Autodesk Inventor part; units mm, degrees
(part 2 of 2)
sketch "Sketch_56" plane through (0, -45.7, 0) normal (0, 1, 0) x (1, 0, 0)
  line L0 (-9.05, 22.27) -> (-9.05, 19.07)
  arc A0 (-9.05, 19.07) -> (-8.65, 18.67) centre (-8.65, 19.07) ccw
  line L1 (-8.65, 18.67) -> (-5.25, 18.67)
  line L2 (-5.25, 18.67) -> (-5.25, 20.67)
  line L3 (-5.25, 20.67) -> (-7.45, 20.67)
  line L4 (-7.45, 20.67) -> (-7.45, 21.67)
  line L5 (-7.45, 21.67) -> (-8.05, 22.67)
  line L6 (-8.05, 22.67) -> (-8.65, 22.67)
  arc A1 (-8.65, 22.67) -> (-9.05, 22.27) centre (-8.65, 22.27) ccw
  constraints: 14 end point, 4 point on circle, 2 centre point
sketch "Sketch_57" plane through (0, 45.9, 0) normal (0, 1, 0) x (1, 0, 0)
  line L0 (-9.05, 22.27) -> (-9.05, 19.07)
  arc A0 (-9.05, 19.07) -> (-8.65, 18.67) centre (-8.65, 19.07) ccw
  line L1 (-8.65, 18.67) -> (-5.25, 18.67)
  line L2 (-5.25, 18.67) -> (-5.25, 20.67)
  line L3 (-5.25, 20.67) -> (-7.45, 20.67)
  line L4 (-7.45, 20.67) -> (-7.45, 21.67)
  line L5 (-7.45, 21.67) -> (-8.05, 22.67)
  line L6 (-8.05, 22.67) -> (-8.65, 22.67)
  arc A1 (-8.65, 22.67) -> (-9.05, 22.27) centre (-8.65, 22.27) ccw
  constraints: 14 end point, 4 point on circle, 2 centre point
sketch "Sketch_62" plane through (-6.25, 0, 0) normal (1, 0, 0) x (0, 0, -1)
  line L0 (-30.83, -44.09) -> (-30.83, -47.3)
  line L1 (-30.83, -47.3) -> (-26.62, -47.3)
  line L2 (-26.62, -47.3) -> (-26.62, -44.09)
  line L3 (-26.62, -44.09) -> (-30.83, -44.09)
  constraints: 8 end point
sketch "Sketch_63" plane through (-6.25, 0, 0) normal (1, 0, 0) x (0, 0, -1)
  line L0 (18.67, -44.09) -> (18.67, -47.3)
  line L1 (18.67, -47.3) -> (22.88, -47.3)
  line L2 (22.88, -47.3) -> (22.88, -44.09)
  line L3 (22.88, -44.09) -> (18.67, -44.09)
  constraints: 8 end point
sketch "Sketch_64" plane through (-6.25, 0, 0) normal (1, 0, 0) x (0, 0, -1)
  line L0 (-30.83, 47.51) -> (-30.83, 44.3)
  line L1 (-30.83, 44.3) -> (-26.62, 44.3)
  line L2 (-26.62, 44.3) -> (-26.62, 47.51)
  line L3 (-26.62, 47.51) -> (-30.83, 47.51)
  constraints: 8 end point
sketch "Sketch_65" plane through (-6.25, 0, 0) normal (1, 0, 0) x (0, 0, -1)
  line L0 (18.67, 47.51) -> (18.67, 44.3)
  line L1 (18.67, 44.3) -> (22.88, 44.3)
  line L2 (22.88, 44.3) -> (22.88, 47.51)
  line L3 (22.88, 47.51) -> (18.67, 47.51)
  constraints: 8 end point
sketch "Sketch_58" plane through (6.25, 0, 0) normal (1, 0, 0) x (0, 0, -1)
  line L0 (18.67, -44.09) -> (18.67, -47.3)
  line L1 (18.67, -47.3) -> (22.88, -47.3)
  line L2 (22.88, -47.3) -> (22.88, -44.09)
  line L3 (22.88, -44.09) -> (18.67, -44.09)
  constraints: 8 end point
extrude "Extrusion53" cut sketch "Sketch_58" along normal mid plane 2
extrude "Extrusion54" cut sketch "Sketch_65" along normal mid plane 2
extrude "Extrusion55" cut sketch "Sketch_64" along normal mid plane 2
extrude "Extrusion56" cut sketch "Sketch_63" along normal mid plane 2
extrude "Extrusion57" cut sketch "Sketch_62" along normal mid plane 2
sketch "Sketch_59" plane through (-6.25, 0, 0) normal (1, 0, 0) x (0, 0, -1)
  circle A0 centre (28.2, 35.1) radius 1.1
  constraints: 1 centre point
sketch "Sketch_66" plane through (-6.25, 0, 0) normal (1, 0, 0) x (0, 0, -1)
  circle A0 centre (-20.3, 40.1) radius 1.1
  constraints: 1 centre point
extrude "Extrusion58" add sketch "Sketch_59" along normal mid plane 2
extrude "Extrusion59" add sketch "Sketch_66" along normal mid plane 2
sketch "Sketch_67" plane through (-6.25, 0, 0) normal (1, 0, 0) x (0, 0, -1)
  circle A0 centre (28.2, -35.1) radius 1.1
  constraints: 1 centre point
sketch "Sketch_68" plane through (-6.25, 0, 0) normal (1, 0, 0) x (0, 0, -1)
  circle A0 centre (-20.3, -40.1) radius 1.1
  constraints: 1 centre point
extrude "Extrusion60" add sketch "Sketch_67" along normal mid plane 2
extrude "Extrusion61" add sketch "Sketch_68" along normal mid plane 2
sketch "Sketch_69" plane through (-2.5, 0, 0) normal (1, 0, 0) x (0, 0, -1)
  line L0 (-51.85, -27.858) -> (-31.85, -27.858)
  line L1 (-31.85, -27.858) -> (-31.85, -27.008)
  line L2 (-31.85, -27.008) -> (-46.85, -27.008)
  line L3 (-46.85, -27.008) -> (-46.85, -12.258)
  line L4 (-46.85, -12.258) -> (-31.85, -12.258)
  line L5 (-31.85, -12.258) -> (-31.85, -11.408)
  line L6 (-31.85, -11.408) -> (-46.85, -11.408)
  line L7 (-46.85, -11.408) -> (-46.85, 3.342)
  line L8 (-46.85, 3.342) -> (-31.85, 3.342)
  line L9 (-31.85, 3.342) -> (-31.85, 4.192)
  line L10 (-31.85, 4.192) -> (-46.85, 4.192)
  line L11 (-46.85, 4.192) -> (-46.85, 18.942)
  line L12 (-46.85, 18.942) -> (-31.85, 18.942)
  line L13 (-31.85, 18.942) -> (-31.85, 19.792)
  line L14 (-31.85, 19.792) -> (-51.85, 19.792)
  line L15 (-51.85, 19.792) -> (-51.85, -27.858)
  constraints: 32 end point
extrude "Extrusion62" cut sketch "Sketch_69" along normal blind 9.5
sketch "Sketch_70" plane through (6.25, 0, 0) normal (1, 0, 0) x (0, 0, -1)
  line L0 (-30.83, 47.51) -> (-30.83, 44.3)
  line L1 (-30.83, 44.3) -> (-26.62, 44.3)
  line L2 (-26.62, 44.3) -> (-26.62, 47.51)
  line L3 (-26.62, 47.51) -> (-30.83, 47.51)
  constraints: 8 end point
extrude "Extrusion63" cut sketch "Sketch_70" along normal mid plane 2
extrude "Extrusion64" add sketch "Sketch_54" along normal mid plane 3.2
extrude "Extrusion65" add sketch "Sketch_55" along normal mid plane 3.2
extrude "Extrusion66" add sketch "Sketch_56" along normal mid plane 3.2
extrude "Extrusion67" add sketch "Sketch_57" along normal mid plane 3.2
body "Solid1"
